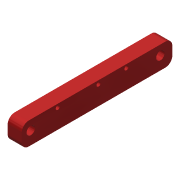
# Autodesk Inventor part: Neje_Base_Slide_y_stop
Saved by Autodesk Inventor 2019.4 (Build 234330000, 330)
## iProperties
Created: 2021-06-27
Part Number: Neje_Base_Slide_y_stop
Material: Generic
Document SubType Name: Modeling
Designer: diederichbenedict
Density: 1 g/cm^3
Appearance: Light Red
Author: diederichbenedict
Autodesk Inventor part; units mm, degrees
ref_plane "YZ Plane" through (0, 0, 0) normal (1, 0, 0) x (0, 1, 0)
ref_plane "XZ Plane" through (0, 0, 0) normal (0, 1, 0) x (-1, 0, 0)
ref_plane "XY Plane" through (0, 0, 0) normal (0, 0, 1) x (1, 0, 0)
sketch "Sketch1" plane through (0, 0.6434, 0) normal (1, 0, 0) x (0, 1, 0)
  circle A0 centre (15.8, 195.0342) radius 3 construction
  circle A1 centre (15.8, 103.0342) radius 3 construction
  circle A2 centre (20.0554, 146.9079) radius 1.45 construction
  circle A3 centre (-24.7132, 132.4283) radius 3.5 construction
  circle A4 centre (-24.9297, 123.6553) radius 3.5 construction
  circle A5 centre (15.1664, 127.0554) radius 4 construction
  circle A6 centre (-25.4429, 102.8495) radius 4 construction
  circle A7 centre (-24.2, 153.2342) radius 4 construction
  circle A8 centre (14.5499, 102.063) radius 2.95 construction
  circle A9 centre (16.8187, 194.035) radius 2.95 construction
  line L0 (-1.4549, 93.9552) -> (-1.2206, 103.4531) construction
  line L1 (-1.4549, 93.9552) -> (16.1397, 93.5212) construction
  arc A10 (16.1397, 93.5212) -> (21.2615, 98.3964) centre (16.263, 98.5197) ccw construction
  line L2 (21.2615, 98.3964) -> (23.652, 195.301) construction
  arc A11 (23.652, 195.301) -> (18.7768, 200.4228) centre (18.6535, 195.4243) ccw construction
  line L3 (18.7768, 200.4228) -> (12.8677, 200.5685) construction
  arc A12 (12.8677, 200.5685) -> (8.4173, 198.0753) centre (12.7444, 195.57) ccw construction
  line L4 (8.4173, 198.0753) -> (0.9275, 185.1387) construction
  line L5 (0.1833, 154.9709) -> (0.9275, 185.1387) construction
  line L6 (-7.9473, 155.1714) -> (0.1833, 154.9709) construction
  line L7 (-7.8733, 158.1705) -> (-7.9473, 155.1714) construction
  line L8 (-2.3058, 158.0332) -> (-7.8733, 158.1705) construction
  line L9 (-1.7513, 180.5119) -> (-2.3058, 158.0332) construction
  line L10 (-1.7513, 180.5119) -> (-12.8987, 161.2579) construction
  line L11 (-29.7936, 161.6747) -> (-12.8987, 161.2579) construction
  arc A13 (-29.7936, 161.6747) -> (-31.8423, 159.7246) centre (-29.8429, 159.6753) ccw construction
  line L12 (-31.8423, 159.7246) -> (-33.3959, 96.7438) construction
  arc A14 (-33.3959, 96.7438) -> (-31.4458, 94.695) centre (-31.3965, 96.6944) ccw construction
  line L13 (-31.4458, 94.695) -> (-3.885, 94.0152) construction
  line L14 (-3.7247, 100.514) -> (-3.885, 94.0152) construction
  line L15 (-9.2922, 100.6513) -> (-3.7247, 100.514) construction
  line L16 (-9.2182, 103.6504) -> (-9.2922, 100.6513) construction
  line L17 (-1.2206, 103.4531) -> (-9.2182, 103.6504) construction
  circle A15 centre (14.1273, 157.9245) radius 4.7908 construction
  line L18 (17.6, 201.4682) -> (11.6, 201.4682)
  line L19 (6.6, 196.4682) -> (6.6, 99.5342)
  line L20 (11.6, 94.5342) -> (17.6, 94.5342)
  line L21 (22.6, 99.5342) -> (22.6, 196.4682)
  arc A16 (11.6, 201.4682) -> (6.6, 196.4682) centre (11.6, 196.4682) ccw
  arc A17 (22.6, 196.4682) -> (17.6, 201.4682) centre (17.6, 196.4682) ccw
  arc A18 (17.6, 94.5342) -> (22.6, 99.5342) centre (17.6, 99.5342) ccw
  arc A19 (6.6, 99.5342) -> (11.6, 94.5342) centre (11.6, 99.5342) ccw
  circle A20 centre (20.0554, 146.9079) radius 1.45 projected
  circle A21 centre (15.8, 103.0342) radius 3 projected
  circle A22 centre (15.8, 195.0342) radius 3 projected
  circle A23 centre (20.198, 175.9006) radius 1.45
  circle A24 centre (20.198, 127.1464) radius 1.45
  point P0 (-0.6434, 0)
  point P1 (6.6, 94.5342)
  dimension "d0" = 16
  dimension "d1" = 5
  dimension "d2" = 2.9
  dimension "d3" = 2.9
  constraints: 8 point on circle, 6 centre point, 6 end point, 6 tangent, 3 equal radius, 2 point on line, 1 horizontal, 1 parallel, 1 perpendicular, 1 vertical, 10 other
  measures "d1" radius of A16
  measures "d2" diameter of A23
  measures "d3" diameter of A24
extrude "Extrusion1" add sketch "Sketch1" along normal blind 10
body "Solid1"
